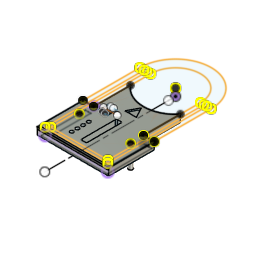
cap (Autodesk Fusion 360 design; units mm, degrees)
Autodesk Fusion 360 part; units mm, degrees
note: some values were not read from the file. Set by a fixed rule: which sketch regions a step uses.
ref_plane "WorkPlane1" through (0, 0, 100) normal (0, 0, 1) x (1, 0, 0)
sketch "Sketch3" plane through (0, 0, 100) normal (0, 0, 1) x (1, 0, 0)
  line L0 (50, -80) -> (50, 0)
  arc A0 (50, 0) -> (-50, 0) centre (0, 0) ccw
  arc A1 (35, 0) -> (-35, 0) centre (0, 0) ccw
  line L1 (35, 0) -> (35, -80)
  line L2 (35, -80) -> (50, -80)
  line L3 (-50, 0) -> (-50, -80)
  line L4 (-50, -80) -> (-35, -80)
  line L5 (-35, -80) -> (-35, 0)
  circle A2 centre (-36, -99) radius 3
  circle A3 centre (36, -99) radius 3
  line L6 (40, -135) -> (-40, -135)
  line L7 (-40, -135) -> (-40, 0)
  line L8 (40, 0) -> (40, -135)
  line L9 (-44, -139) -> (-44, 0)
  line L10 (44, 0) -> (44, -139)
  line L11 (44, -139) -> (-44, -139)
  arc A4 (-35, -28.2843) -> (35, -28.2843) centre (0, 0) ccw
  line L12 (-35, -28.2843) -> (-35, -80)
  line L13 (-50, -80) -> (-50, -144)
  line L14 (-50, -144) -> (50, -144)
  line L15 (50, -144) -> (50, -80)
  line L16 (50, -80) -> (35, -80)
  line L17 (35, -28.2843) -> (35, -80)
  line L18 (-50, -80) -> (-35, -80)
  circle A5 centre (-36, -99) radius 2.8
  circle A6 centre (36, -99) radius 2.9
  dimension "d2" = 90
  dimension "d3" = 5.6
  dimension "d4" = 5.8
  dimension "d15" = 64
  constraint concentric A1 A4
  constraint coincident L5 A4.start
  constraint coincident L1 A4.end
  constraint coincident L4.end L5.start
  constraint coincident L3.end L4.start
  constraint perpendicular L11 L13
  constraint perpendicular L10 L14
  constraint coincident L0.start L2.end
  constraint perpendicular L14 L15
  constraint coincident L1.end L2.start
  constraint concentric A2 A5
  constraint concentric A3 A6
  measures "d2" diameter of A4
  measures "d3" diameter of A5
  measures "d4" diameter of A6
  measures "d15" distance of L14.end L0.start
extrude "Extrude1" add sketch "Sketch3" against normal blind 10 contours L2 L4 L9 L10 L11 L13 L14 L15 L16 L18 | L2 L4 L6 L7 L8 L9 L10 L11 L16 L18 | L1 L2 L4 L5 L6 L7 L8 A4 L12 L16 L17 L18 makes body 1
extrude "Extrude2" add sketch "Sketch3" against normal blind 30 separate body contours A5 | A6 makes body 2 at (-33.541, -100.3391, 80) makes body 3 at (37.1927, -96.3566, 80)
sketch "Sketch6" plane through (0, 0, 90) normal (0, 0, -1) x (1, 0, 0)
  circle A0 centre (36, 99) radius 3
  circle A1 centre (-36, 99) radius 3
  line L0 (50, 144) -> (-50, 144)
  line L1 (-50, 144) -> (-50, 80)
  line L2 (-50, 80) -> (-35, 80)
  line L3 (-35, 80) -> (-35, 28.2843)
  arc A2 (35, 28.2843) -> (-35, 28.2843) centre (0, 0) ccw
  line L4 (35, 28.2843) -> (35, 80)
  line L5 (35, 80) -> (50, 80)
  line L6 (50, 80) -> (50, 144)
  line L7 (35, 80) -> (42.5, 80)
  line L8 (42.5, 80) -> (46.5, 80)
  line L9 (42.5, 80) -> (39, 80)
  line L10 (46.5, 80) -> (46.5, 133)
  line L11 (39, 80) -> (39, 132)
  line L12 (0, 0) -> (0, 10)
  line L13 (0, 10) -> (0, 183.5284)
  line L14 (0, 10) -> (0, 183.5284)
  line L15 (-39, 80) -> (-39, 132)
  line L16 (-46.5, 80) -> (-46.5, 133)
  line L17 (-42.5, 80) -> (-39, 80)
  line L18 (-42.5, 80) -> (-46.5, 80)
  line L19 (-39, 132) -> (39, 132)
  line L20 (46.5, 133) -> (46.5, 142)
  line L21 (-46.5, 133) -> (-46.5, 142)
  line L22 (-46.5, 142) -> (46.5, 142)
  line L23 (44, 139) -> (-44, 139)
  dimension "d9" = 4
  dimension "d10" = 3.5
  dimension "d11" = 53
  dimension "d12" = 52
  dimension "d19" = 3
  constraint coincident L4.end L5.start
  constraint midpoint L5 L7.end
  constraint parallel L5 L8
  constraint parallel L7 L9
  constraint perpendicular L8 L10
  constraint perpendicular L9 L11
  constraint coincident A2.centre L12.start
  constraint vertical L12
  constraint parallel L12 L13
  constraint symmetric L7.end L13 L17.start
  constraint symmetric L8.end L13 L16.start
  constraint symmetric L9.end L13 L15.start
  constraint symmetric L10.end L13 L16.end
  constraint symmetric L11.end L13 L15.end
  constraint symmetric L12.end L13 L14.start
  constraint symmetric L14.end L13 L13.end
  constraint parallel L10 L20
  constraint parallel L16 L21
  constraint perpendicular L20 L22
  measures "d9" distance of L7.end L8.end
  measures "d10" distance of L7.end L9.end
  measures "d11" distance of L8.end L10.end
  measures "d12" distance of L9.end L11.end
  measures "d19" distance of L22 L23
extrude "Extrude4" cut sketch "Sketch6" against normal blind 4 contours L5 L7 L8 L9 L10 L11 L13 L14 L19 L20 L22 | L2 L13 L14 L15 L16 L17 L18 L19 L21 L22 bodies 1
sketch "Sketch7" plane through (0, 0, 100) normal (0, 0, 1) x (1, 0, 0)
  line L0 (-20, -101.7213) -> (-20, -125.7213)
  circle A0 centre (-20, -101.7213) radius 2.5
  circle A1 centre (-20, -125.7213) radius 2.5
  circle A2 centre (-20, -117.7213) radius 2.5
  circle A3 centre (-20, -109.7213) radius 2.5
  dimension "d20" = 5
  dimension "d21" = 24
  dimension "d22" = 5
  dimension "d23" = 5
  dimension "d24" = 5
  dimension "d28" = 8
  dimension "d30" = 8
  dimension "d31" = 8
  constraint vertical L0
  constraint coincident L0.start A0.centre
  constraint coincident L0.end A1.centre
  constraint coincident L0 A2.centre
  constraint coincident L0 A3.centre
  measures "d20" diameter of A0
  measures "d21" distance of L0.start L0.end
  measures "d22" diameter of A1
  measures "d23" diameter of A2
  measures "d24" diameter of A3
  measures "d28" distance of L0.start A3.centre
  measures "d30" distance of A2.centre A3.centre
  measures "d31" distance of L0.end A2.centre
extrude "Extrude5" cut sketch "Sketch7" against normal blind 45 bodies 1
sketch "Sketch8" plane through (0, 0, 100) normal (0, 0, 1) x (1, 0, 0)
  line L0 (-27, -68.082) -> (-14.9, -68.082)
  line L1 (-14.9, -68.082) -> (-14.9, -80.182)
  line L2 (-14.9, -80.182) -> (-27, -80.182)
  line L3 (-27, -80.182) -> (-27, -68.082)
  line L4 (-27, -80.182) -> (-23, -80.182)
  circle A0 centre (-23, -80.182) radius 1
  line L5 (-23, -80.182) -> (-19, -80.182)
  circle A1 centre (-19, -80.182) radius 1
  line L6 (-27, -68.082) -> (-27, -74.082)
  line L7 (-27, -74.082) -> (-7.7924, -74.082)
  line L8 (-27, -74.082) -> (-7.7924, -74.082)
  circle A2 centre (-23, -67.982) radius 1
  circle A3 centre (-19, -67.982) radius 1
  point P0 (-35, -80)
  dimension "d34" = 12.1
  dimension "d35" = 12.1
  dimension "d36" = 4
  dimension "d37" = 2
  dimension "d38" = 4
  dimension "d39" = 2
  dimension "d40" = 6
  dimension "d41" = 8
  constraint horizontal L0
  constraint vertical L1
  constraint horizontal L2
  constraint vertical L3
  constraint perpendicular L3 L4
  constraint coincident L4.end A0.centre
  constraint parallel L2 L5
  constraint coincident L5.end A1.centre
  constraint perpendicular L0 L6
  constraint perpendicular L1 L7
  constraint symmetric A0 L7 A2
  constraint symmetric A1 L7 A3
  constraint symmetric L6.end L7 L8.start
  constraint symmetric L8.end L7 L7.end
  measures "d34" distance of L0.start L0.end
  measures "d35" distance of L0.start L2.end
  measures "d36" distance of L2.end L4.end
  measures "d37" diameter of A0
  measures "d38" distance of L4.end L5.end
  measures "d39" diameter of A1
  measures "d40" distance of L0.start L6.end
  measures "d41" horizontal distance of L2.end P0
extrude "Extrude6" cut sketch "Sketch8" against normal blind 17 contours L0 A2 | L0 A2 | L0 A3 | L0 A3 | L2 L4 A0 L5 | L2 L4 A0 L5 | L2 L5 A1 | L2 L5 A1 bodies 1
extrude "Extrude7" cut sketch "Sketch8" against normal blind 7 contours L0 L1 L3 L6 L7 L8 A2 A3 | L1 L2 L3 L4 A0 L5 A1 L7 L8 bodies 1
sketch "Sketch9" plane through (0, 0, 100) normal (0, 0, 1) x (1, 0, 0)
  line L0 (4, -79) -> (-4, -79)
  line L1 (-4, -79) -> (-4, -129)
  line L2 (-4, -129) -> (4, -129)
  line L3 (4, -129) -> (4, -79)
  line L4 (4, -79) -> (-4, -129) construction
  line L5 (-4, -79) -> (4, -129) construction
  line L6 (-50, -144) -> (50, -144)
  point P0 (0, -104)
  dimension "d46" = 8
  dimension "d47" = 50
  dimension "d48" = 15
  constraint horizontal L0
  constraint perpendicular L0 L1
  constraint parallel L0 L2
  constraint parallel L1 L3
  constraint coincident L4 P0
  constraint coincident L5 P0
  measures "d46" distance of L1.end L2.end
  measures "d47" distance of L0.end L1.end
  measures "d48" distance of L2 L6
extrude "Extrude8" cut sketch "Sketch9" against normal blind 55 bodies 1
fillet "Fillet1" radius 1.5 4 edges at (-4, -79, 95) (4, -79, 95) (-4, -129, 95) (4, -129, 95) on bodies 1
fillet "Fillet2" radius 3 1 edges at (0, -144, 100) on bodies 1
sketch "Sketch12" plane through (0, 0, 100) normal (0, 0, 1) x (1, 0, 0)
  line L0 (0, -63) -> (8, -63)
  line L1 (0, -63) -> (-8, -63)
  line L2 (-8, -63) -> (-0.019, -47.9899)
  line L3 (-8, -63) -> (4.6601, -63) construction
  line L4 (0, -10) -> (0, -183.5284)
  line L5 (-0.019, -47.9899) -> (7.962, -63)
  line L6 (-0.019, -47.9899) -> (16.981, -47.9899) construction
  dimension "d78" = 8
  dimension "d79" = 8
  dimension "d80" = 17
  dimension "d81" = 62
  dimension "d82" = 17
  dimension "d83" = 62
  constraint horizontal L0
  constraint parallel L0 L1
  constraint horizontal L3
  constraint coincident L0.start L4
  constraint horizontal L6
  measures "d78" distance of L0.start L0.end
  measures "d79" distance of L0.start L1.end
  measures "d80" distance of L1.end L2.end
  measures "d81" angle of L2 L3
  measures "d82" distance of L2.end L5.end
  measures "d83" angle of L5 L6
extrude "Extrude10" cut sketch "Sketch12" against normal blind 2 bodies 1
equation "d7 = -23 mm - 7 mm"
